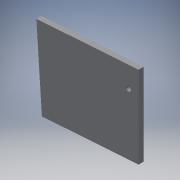
# Autodesk Inventor part: 2018 Intake Plate
Saved by Autodesk Inventor 2018 (Build 220112000, 112)
## iProperties
Created: 2018-01-28
Part Number: 2018 Intake Plate
Material: Generic
Document SubType Name: Modeling
Designer: Apple
Density: 1 g/cm^3
Appearance: Default
Author: Apple
Autodesk Inventor part; units mm, degrees
ref_plane "YZ Plane" through (0, 0, 0) normal (1, 0, 0) x (0, 1, 0)
ref_plane "XZ Plane" through (0, 0, 0) normal (0, 1, 0) x (-1, 0, 0)
ref_plane "XY Plane" through (0, 0, 0) normal (0, 0, 1) x (1, 0, 0)
sketch "Sketch1" plane through (0, 0, 0) normal (0, 0, 1) x (1, 0, 0)
  circle A0 centre (12.7, 635.3302) radius 3.175 projected
  circle A1 centre (12.7, 635.3302) radius 3.175 projected
  circle A2 centre (12.7, 723.9) radius 6.35 projected
  circle A3 centre (12.7, 12.7) radius 6.35 projected
  circle A4 centre (12.7, 368.3) radius 6.35 projected
  line L0 (25.4, 0) -> (0, 0) projected
  line L1 (0, 0) -> (0, 736.6) projected
  line L2 (25.4, 736.6) -> (0, 736.6) projected
  line L3 (25.4, 0) -> (25.4, 736.6) projected
  line L4 (25.4, 661.652) -> (-101.3077, 653.0401)
  line L5 (-101.3077, 653.0401) -> (-94.4182, 551.6739)
  line L6 (-94.4182, 551.6739) -> (25.4, 559.8176)
  line L7 (25.4, 661.652) -> (25.4, 559.8176)
  circle A5 centre (12.7, 635.3302) radius 3.175
  dimension "d0" = 101.6
  dimension "d1" = 127
  dimension "d2" = 25.4
  constraints: 8 end point, 2 perpendicular, 2 point on line, 1 centre point, 1 coincident, 1 collinear, 1 concentric
  measures "d0" distance of L4.end L5.end
  measures "d1" distance of L4.start L4.end
  measures "d2" distance from line of L4 A0.centre
extrude "Extrusion1" add sketch "Sketch1" along normal blind 6.35 contours L6 L1 L4 L3 | L6 L5 L4 L1
sketch "Sketch2" plane through (0, 0, 0) normal (0, 0, -1) x (-1, 0, 0)
  circle A0 centre (37.4278, 642.601) radius 12.7 projected
  point P0 (0, 0)
extrude "Extrusion2" cut sketch "Sketch2" against normal through all
body "Solid1"
